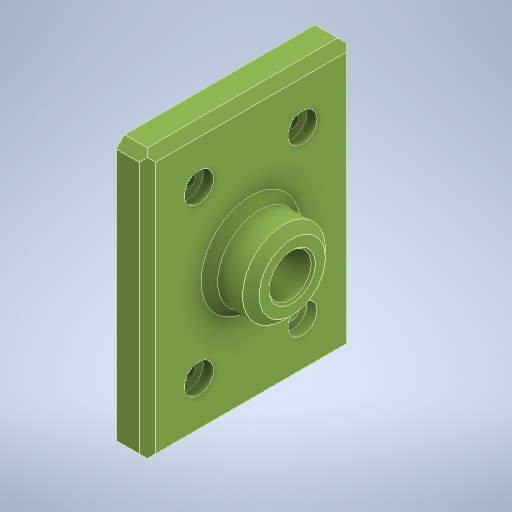
# Autodesk Inventor part: Front_Cover
Saved by Autodesk Inventor 2026.2 (Build 302298010, 298A)
## iProperties
Created: 2026-05-07
Part Number: Front_Cover
Material: Generic
Document SubType Name: Modeling
Designer: piete
Density: 1 g/cm^3
Appearance: Olive Green
Author: piete
Autodesk Inventor part; units mm, degrees
ref_plane "YZ Plane" through (0, 0, 0) normal (1, 0, 0) x (0, 1, 0)
ref_plane "XZ Plane" through (0, 0, 0) normal (0, 1, 0) x (-1, 0, 0)
ref_plane "XY Plane" through (0, 0, 0) normal (0, 0, 1) x (1, 0, 0)
sketch "Sketch1" plane through (0, 0, 0) normal (1, 0, 0) x (0, 1, 0)
  line L0 (32.5, 25) -> (-32.5, 25)
  line L1 (-32.5, 25) -> (-32.5, -25)
  line L2 (-32.5, -25) -> (32.5, -25)
  line L3 (32.5, -25) -> (32.5, 25)
  point P0 (0, 0)
  dimension "d0" = 65
  dimension "d1" = 50
  dimension "d2" = 32.5
  dimension "d3" = 25
  constraints: 8 end point, 2 parallel, 1 horizontal, 1 perpendicular
  measures "d0" distance of L2.end L1.end
  measures "d1" distance of L1.end L0.end
  measures "d2" distance from line of point (0, 0) L3
  measures "d3" distance from line of L0 point (0, 0)
extrude "Extrusion1" add sketch "Sketch1" along normal blind 7.5
sketch "Sketch2" plane through (7.5, 0, 0) normal (1, 0, 0) x (0, 0, -1)
  circle A0 centre (-12.5, 20) radius 1.6
  line L0 (25, 32.5) -> (-25, 32.5) projected
  line L1 (-25, 32.5) -> (-25, -32.5) projected
  circle A1 centre (12.5, 20) radius 1.6
  line L2 (25, -32.5) -> (25, 32.5) projected
  point P0 (0, 0)
  dimension "d6" = 3.2
  dimension "d7" = 12.5
  dimension "d8" = 12.5
  dimension "d9" = 3.2
  dimension "d10" = 12.5
  dimension "d11" = 12.5
  constraints: 2 centre point
  measures "d6" diameter of A0
  measures "d7" distance from line of L0 A0.centre
  measures "d8" distance from line of L1 A0.centre
  measures "d9" diameter of A1
  measures "d10" distance from line of L0 A1.centre
  measures "d11" distance from line of L2 A1.centre
extrude "Extrusion2" cut sketch "Sketch2" against normal through all
sketch "Sketch3" plane through (7.5, 0, 0) normal (1, 0, 0) x (0, 0, -1)
  circle A0 centre (0, 0) radius 10
  dimension "d14" = 20
  constraints: 1 centre point, 1 coincident
  measures "d14" diameter of A0
extrude "Extrusion3" add sketch "Sketch3" along normal blind 10
sketch "Sketch4" plane through (17.5, 0, 0) normal (1, 0, 0) x (0, 0, -1)
  circle A0 centre (0, 0) radius 5.1
  dimension "d17" = 10.2
  constraints: 1 centre point, 1 coincident
  measures "d17" diameter of A0
extrude "Extrusion4" cut sketch "Sketch4" against normal through all draft -0.75
chamfer "Chamfer1" distance 2 angle 45 6 edges at (7.5, 0, 10) (17.5, 0, 10) (7.5, 0, 25) (7.5, 32.5, 0) (7.5, 0, -25) (7.5, -32.5, 0)
chamfer "Chamfer2" distance 0.5 angle 45 1 edges at (17.5, 0, 5.1)
mirror "Mirror1" about plane through (0, 0, 0) normal (0, 1, 0) of "Extrusion2"
chamfer "Chamfer3" distance 2 angle 45 4 edges at (2.75, 32.5, 25) (2.75, 32.5, -25) (2.75, -32.5, 25) (2.75, -32.5, -25)
sketch "Sketch5" plane through (7.5, 0, 0) normal (1, 0, 0) x (0, 0, -1)
  circle A0 centre (-12.5, 20) radius 1.6 projected
  circle A1 centre (-12.5, 20) radius 3.5
  circle A2 centre (12.5, 20) radius 1.6 projected
  circle A3 centre (12.5, 20) radius 3.5
  circle A4 centre (12.5, -20) radius 1.6 projected
  circle A5 centre (12.5, -20) radius 3.5
  circle A6 centre (-12.5, -20) radius 1.6 projected
  circle A7 centre (-12.5, -20) radius 3.5
  point P0 (0, 0)
  dimension "d29" = 7
  dimension "d30" = 7
  dimension "d31" = 7
  dimension "d32" = 7
  constraints: 4 centre point, 4 coincident
  measures "d29" diameter of A1
  measures "d30" diameter of A3
  measures "d31" diameter of A5
  measures "d32" diameter of A7
extrude "Extrusion5" cut sketch "Sketch5" against normal blind 2.5 contours A0 | A1 | A2 | A3 | A4 | A5 | A6 | A7
equation "\"d2\" = 0.5 * d0"
equation "\"d3\" = 0.5 * d1"
body "Solid1"
